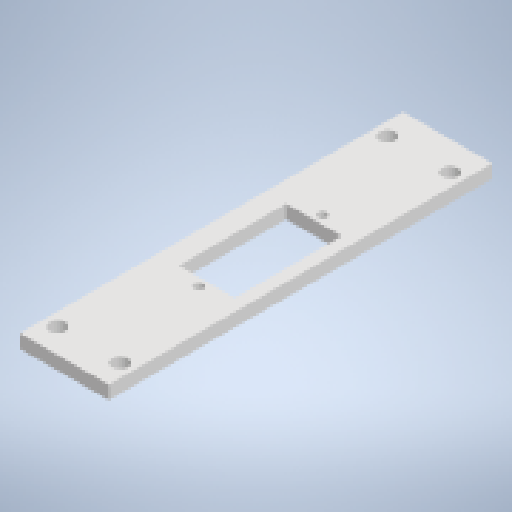
# Autodesk Inventor part: support_servo_moteur
Saved by Autodesk Inventor 2024 (Build 280153000, 153)
## iProperties
Created: 2021-11-10
Part Number: support_servo_moteur
Material: Générique
Document SubType Name: Modeling
Designer: ropertth
Density: 1 g/cm^3
Appearance: Par défaut
Mass: 4.1257 g
Surface Area: 37.7511 cm^2
Volume: 4.1257 cm^3
Author: ropertth
Autodesk Inventor part; units mm, degrees
ref_plane "YZ Plane" through (0, 0, 0) normal (1, 0, 0) x (0, 1, 0)
ref_plane "XZ Plane" through (0, 0, 0) normal (0, 1, 0) x (-1, 0, 0)
ref_plane "XY Plane" through (0, 0, 0) normal (0, 0, 1) x (1, 0, 0)
sketch "Esquisse1" plane through (0, 0, 0) normal (0, 1, 0) x (-1, 0, 0)
  line L0 (0, 0) -> (20, 0)
  line L1 (20, 0) -> (20, -86)
  line L2 (20, -86) -> (0, -86)
  line L3 (0, -86) -> (0, 0)
  dimension "d0" = 86
  dimension "d1" = 20
  constraints: 8 end point, 2 parallel, 1 horizontal, 1 perpendicular
  measures "d0" distance of L0.end L1.end
  measures "d1" distance of L0.start L0.end
extrude "Extrusion1" add sketch "Esquisse1" along normal blind 3
sketch "Esquisse2" plane through (0, 3, 0) normal (0, 1, 0) x (1, 0, 0)
  line L0 (-20, 0) -> (0, 0) projected
  line L1 (0, 0) -> (0, 86) projected
  line L2 (10.8927, 42.5) -> (-28.8955, 42.5) construction
  point P0 (-3, 6)
  dimension "d12" = 3
  dimension "d37" = 42.5
  dimension "d39" = 36.5
  constraints: 2 end point, 1 horizontal
  measures "d12" distance from line of L1 point (-3, 6)
  measures "d37" distance between parallel lines of L0 L2
  measures "d39" distance from line of L2 point (-3, 6)
hole "Perçage1" at (-3, 3, -6) direction (0, -1, 0) diameter 3.5 end through all
pattern_linear "Réseau rectangulaire1" count 2 spacing 14 along (-1, 0, 0) count 2 spacing 74 along (0, 0, -1) of "Perçage1"
sketch "Esquisse3" plane through (0, 3, 0) normal (0, 1, 0) x (1, 0, 0)
  line L0 (-15.25, 31) -> (-2.75, 31)
  line L1 (-2.75, 31) -> (-2.75, 55)
  line L2 (-2.75, 55) -> (-15.25, 55)
  line L3 (-15.25, 55) -> (-15.25, 31)
  line L4 (0, 86) -> (-20, 86) projected
  line L5 (-20, 86) -> (-20, 0) projected
  point P0 (0, 0)
  dimension "d19" = 24
  dimension "d20" = 12.5
  dimension "d21" = 31
  dimension "d22" = 4.75
  constraints: 8 end point, 2 parallel, 1 horizontal, 1 perpendicular
  measures "d19" distance of L2.end L0.start
  measures "d20" distance of L1.end L2.end
  measures "d21" distance between parallel lines of L4 L2
  measures "d22" distance between parallel lines of L5 L3
extrude "Extrusion2" cut sketch "Esquisse3" against normal through all
sketch "Esquisse4" plane through (0, 3, 0) normal (0, 1, 0) x (1, 0, 0)
  line L0 (-2.75, 55) -> (-2.75, 31) projected
  line L1 (-2.75, 31) -> (-15.25, 31) projected
  point P0 (0, 0)
  point P1 (-9, 29.15)
  dimension "d32" = 6.25
  dimension "d33" = 1.85
  measures "d32" distance from line of L0 point (-9, 29.15)
  measures "d33" distance from line of L1 point (-9, 29.15)
hole "Perçage2" at (-9, 3, -29.15) direction (0, -1, 0) diameter 2 end through all
pattern_linear "Réseau rectangulaire2" count 2 spacing 27.7 along (0, 0, -1) of "Perçage2"
